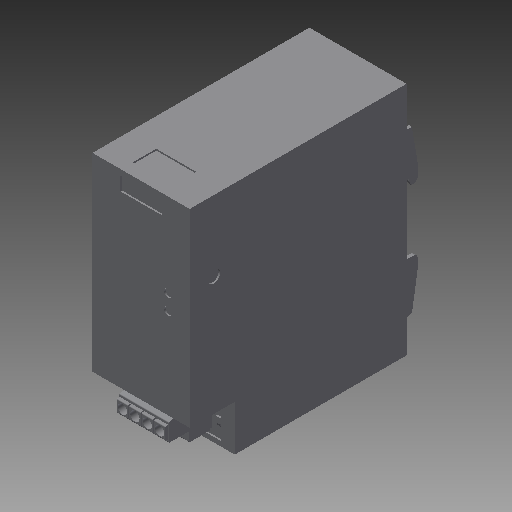
# Autodesk Inventor part: 172882
Saved by Autodesk Inventor 2019.3 (Build 233278000, 278)
## iProperties
Category: PARTsolutions
Company: MOELLER
Created: 2018-10-25
Part Number: 172882
Material: Generic
Catalog Web Link: www.cadenas.de
Description: PSG Power supply units-
Vendor: MOELLER
Document SubType Name: Modeling
Designer: psadmin
Manufacturer: MOELLER
Mass: 656.028 g
Surface Area: 554.305 cm^2
Volume: 656.028 cm^3
Density: 1 g/cm^3
Appearance: PSOLRGB-175-175-175
PSOL_IDENT_0: {$CADENAS_DATA\23d-libs\moeller\1589\1805\1806.prj},181 {VTYP=3D},{NB=172882},{LINA=172882},{NN=PSG
PSOL_IDENT_1: Power supply units},{DATE=04.10.2018 12:16:39},{GEOMDATE=04.10.2018 08:29:25},{VERSION=v181004082925
PSOL_IDENT_2: },{LINEID=10},{WBVAR=},{WBNUMERIC=}  {NB=172882},{LINA=172882},{KT=DUMMY},{PFOTO=2727pic-70.jpg},{PL
PSOL_IDENT_3: ID=172882},{DATA_SHEET=Data sheet},{MANUTYPEDESC=PSG60F24RM},{DESCSHORT=Power supply unit, 3-phase,
PSOL_IDENT_4: 100-240VAC/24VDC, 2.5A},{DESCLONG=Power supply unit, Product range: Power supplies PSG, Subrange: po
PSOL_IDENT_5: wer supply unit, Description: Power Boost via 1.5-fold rated operational current for 5 s, PELV (EN 6
PSOL_IDENT_6: 0204), SELV (EN 60950), Width: 50 mm, Height: 121 mm, Depth: 117.3 mm, Three-phase, Input voltage ra
PSOL_IDENT_7: nge: 320 - 600 V AC, (450 - 800 V DC), Nominal input voltage: 3 x 400 - 500 V AC, Rated output volta
PSOL_IDENT_8: ge: 24 V DC (± 2%), Rated output current: 2.5 A, Setting range for the output voltage: 24 - 28 V DC,
PSOL_IDENT_9: Rated output power: 60 W, Degree of Protection: IP20, Heat dissipation: 9.8 W},{EAN=4015081694709},
PSOL_IDENT_10: {ECLASS_8_1=27-04-90-02},{PACKAGED_WEIGHT=0.610},{DATA_SHEET_=http://datasheet.moeller.net/datasheet
PSOL_IDENT_11: .php?model=172882&locale=en_GB},{DATA_SHEET_ENG=http://datasheet.moeller.net/datasheet.php?model=172
PSOL_IDENT_12: 882&locale=en_GB},{DATA_SHEET_DEU=http://datasheet.moeller.net/datasheet.php?model=172882&locale=de_
PSOL_IDENT_13: DE}
NN: PSG Power supply units
NB: 172882
NBSYN: $PLID.
LINA: 172882
PFOTO: 2727pic-70.jpg
PLID: 172882
DATA_SHEET: Data sheet
MANUTYPEDESC: PSG60F24RM
DESCSHORT: Power supply unit, 3-phase, 100-240VAC/24VDC, 2.5A
DESCLONG: Power supply unit, Product range: Power supplies PSG, Subrange: power supply unit, Description: Power Boost via 1.5-fold rated operational current for 5 s, PELV (EN 60204), SELV (EN 60950), Width: 50 mm, Height: 121 mm, Depth: 117.3 mm, Three-phase, Input voltage range: 320 - 600 V AC, (450 - 800 V DC), Nominal input voltage: 3 x 400 - 500 V AC, Rated output voltage: 24 V DC (± 2%), Rated output current: 2.5 A, Setting range for the output voltage: 24 - 28 V DC, Rated output power: 60 W, Degree of Protection: IP20, Heat dissipation: 9.8 W
EAN: 4015081694709
ECLASS_8_1: 27-04-90-02
PACKAGED_WEIGHT: 0.61
SUPPLIER: MOELLER
ARTICLENO: 172882
BOMINFO: 172882
CREATOR: CADENAS GmbH
Title: 172882
Author: Cadenas PARTsolutions
Autodesk Inventor part; units mm, degrees
ref_plane "YZ Plane" through (0, 0, 0) normal (1, 0, 0) x (0, 1, 0)
ref_plane "XZ Plane" through (0, 0, 0) normal (0, 1, 0) x (-1, 0, 0)
ref_plane "XY Plane" through (0, 0, 0) normal (0, 0, 1) x (1, 0, 0)
sketch "Sketch_1" plane through (0, 0, 0) normal (1, 0, 0) x (0, 1, 0)
  line L0 (23.5, 23.2) -> (23.5, 0)
  line L1 (23.5, 0) -> (0, 0)
  line L2 (0, 0) -> (0, -88.4)
  line L3 (0, -88.4) -> (17, -88.4)
  line L4 (17, -88.4) -> (17, -89.3953)
  arc A0 (17, -89.3953) -> (18.6832, -91.37) centre (19, -89.3953) ccw
  line L5 (18.6832, -91.37) -> (35.7, -94.1)
  line L6 (35.7, -94.1) -> (40.7, -94.1)
  arc A1 (40.7, -94.1) -> (42.7, -92.1) centre (40.7, -92.1) ccw
  line L7 (42.7, -92.1) -> (42.7, -88.4)
  line L8 (42.7, -88.4) -> (78, -88.4)
  line L9 (78, -88.4) -> (78, -89.7)
  line L10 (78, -89.7) -> (77, -89.7)
  line L11 (77, -89.7) -> (74.7, -90.773)
  line L12 (74.7, -90.773) -> (74.7, -92.1)
  arc A2 (74.7, -92.1) -> (76.7, -94.1) centre (76.7, -92.1) ccw
  line L13 (76.7, -94.1) -> (83, -94.1)
  line L14 (83, -94.1) -> (100.5, -91.1)
  line L15 (100.5, -91.1) -> (100.5, -88.4)
  line L16 (100.5, -88.4) -> (121, -88.4)
  line L17 (121, -88.4) -> (121, 23.2)
  line L18 (121, 23.2) -> (23.5, 23.2)
  constraints: 38 end point, 6 point on circle, 3 centre point
extrude "Extrusion1" add sketch "Sketch_1" along normal blind 50
sketch "Sketch_2" plane through (0, 0, 0) normal (0, 1, 0) x (-1, 0, 0)
  line L0 (-1.6, -98.4) -> (-1.6, -88.4)
  line L1 (-1.6, -88.4) -> (-48.4, -88.4)
  line L2 (-48.4, -88.4) -> (-48.4, -98.4)
  line L3 (-48.4, -98.4) -> (-1.6, -98.4)
  constraints: 8 end point
extrude "Extrusion2" cut sketch "Sketch_2" along normal blind 120
sketch "Sketch_9" plane through (0, 0, 0) normal (0, 0, 1) x (1, 0, 0)
  line L0 (5.65, 22.3) -> (8.85, 22.3)
  line L1 (8.85, 22.3) -> (9.85, 21.3)
  line L2 (9.85, 21.3) -> (9.85, 18)
  line L3 (9.85, 18) -> (7.85, 18)
  line L4 (7.85, 18) -> (7.85, 19.5)
  arc A0 (7.85, 19.5) -> (6.85, 19.5) centre (7.35, 19.5) ccw
  line L5 (6.85, 19.5) -> (6.85, 12.5)
  line L6 (6.85, 12.5) -> (9.85, 12.5)
  line L7 (9.85, 12.5) -> (9.85, 8)
  line L8 (9.85, 8) -> (7.85, 8)
  line L9 (7.85, 8) -> (7.85, 9.5)
  arc A1 (7.85, 9.5) -> (6.85, 9.5) centre (7.35, 9.5) ccw
  line L10 (6.85, 9.5) -> (6.85, 2.5)
  line L11 (6.85, 2.5) -> (43.15, 2.5)
  line L12 (43.15, 2.5) -> (43.15, 9.5)
  arc A2 (43.15, 9.5) -> (42.15, 9.5) centre (42.65, 9.5) ccw
  line L13 (42.15, 9.5) -> (42.15, 8)
  line L14 (42.15, 8) -> (40.15, 8)
  line L15 (40.15, 8) -> (40.15, 12.5)
  line L16 (40.15, 12.5) -> (43.15, 12.5)
  line L17 (43.15, 12.5) -> (43.15, 19.5)
  arc A3 (43.15, 19.5) -> (42.15, 19.5) centre (42.65, 19.5) ccw
  line L18 (42.15, 19.5) -> (42.15, 18)
  line L19 (42.15, 18) -> (40.15, 18)
  line L20 (40.15, 18) -> (40.15, 21.3)
  line L21 (40.15, 21.3) -> (41.15, 22.3)
  line L22 (41.15, 22.3) -> (44.35, 22.3)
  line L23 (44.35, 22.3) -> (44.35, 23.484)
  line L24 (44.35, 23.484) -> (5.65, 23.484)
  line L25 (5.65, 23.484) -> (5.65, 22.3)
  line L26 (12.3, 20.65) -> (12.3, 5.6)
  line L27 (12.3, 5.6) -> (37.7, 5.6)
  line L28 (37.7, 5.6) -> (37.7, 20.65)
  line L29 (37.7, 20.65) -> (12.3, 20.65)
  constraints: 60 end point, 8 point on circle, 4 centre point
extrude "Extrusion3" cut sketch "Sketch_9" against normal blind 0.8
sketch "Sketch_10" plane through (25, 0, 0) normal (1, 0, 0) x (0, 0, -1)
  line L0 (0, 19.5) -> (0, 18)
  line L1 (0, 18) -> (0.8, 18)
  line L2 (0.8, 18) -> (0, 19.5)
  constraints: 6 end point
extrude "Extrusion4" cut sketch "Sketch_10" along normal mid plane 36
sketch "Sketch_11" plane through (25, 0, 0) normal (1, 0, 0) x (0, 0, -1)
  line L0 (0, 9.5) -> (0, 8)
  line L1 (0, 8) -> (0.8, 8)
  line L2 (0.8, 8) -> (0, 9.5)
  constraints: 6 end point
extrude "Extrusion5" cut sketch "Sketch_11" along normal mid plane 36
sketch "Sketch_12" plane through (25, 0, 0) normal (1, 0, 0) x (0, 0, -1)
  line L0 (0, 9.5) -> (0, 8)
  line L1 (0, 8) -> (0.8, 8)
  line L2 (0.8, 8) -> (0, 9.5)
  constraints: 6 end point
extrude "Extrusion6" add sketch "Sketch_12" along normal mid plane 25.4
sketch "Sketch_13" plane through (25, 0, 0) normal (1, 0, 0) x (0, 0, -1)
  line L0 (0, 19.5) -> (0, 18)
  line L1 (0, 18) -> (0.8, 18)
  line L2 (0.8, 18) -> (0, 19.5)
  constraints: 6 end point
extrude "Extrusion7" add sketch "Sketch_13" along normal mid plane 25.4
sketch "Sketch_3" plane through (25, 0, 0) normal (1, 0, 0) x (0, 0, -1)
  line L0 (-23.2, 17.3) -> (-23.2, 11.8)
  arc A0 (-23.2, 11.8) -> (-22.7, 11.3) centre (-22.7, 11.8) ccw
  line L1 (-22.7, 11.3) -> (-21.7, 11.3)
  line L2 (-21.7, 11.3) -> (-21.7, 10.3)
  arc A1 (-21.7, 10.3) -> (-21.2, 9.8) centre (-21.2, 10.3) ccw
  line L3 (-21.2, 9.8) -> (-11.25, 9.8)
  line L4 (-11.25, 9.8) -> (-11.25, 5.3)
  arc A2 (-11.25, 5.3) -> (-10.75, 4.8) centre (-10.75, 5.3) ccw
  line L5 (-10.75, 4.8) -> (-0.25, 4.8)
  line L6 (-0.25, 4.8) -> (-0.25, 5.6)
  line L7 (-0.25, 5.6) -> (0, 5.6)
  line L8 (0, 5.6) -> (0, 20.65)
  line L9 (0, 20.65) -> (-11.25, 20.65)
  line L10 (-11.25, 20.65) -> (-21.272, 19.1912)
  arc A3 (-21.272, 19.1912) -> (-21.7, 18.6964) centre (-21.2, 18.6964) ccw
  line L11 (-21.7, 18.6964) -> (-21.7, 17.8)
  line L12 (-21.7, 17.8) -> (-22.7, 17.8)
  arc A4 (-22.7, 17.8) -> (-23.2, 17.3) centre (-22.7, 17.3) ccw
  constraints: 26 end point, 10 point on circle, 5 centre point
extrude "Extrusion8" add sketch "Sketch_3" along normal mid plane 25.4
sketch "Sketch_4" plane through (0, 0, 0) normal (0, 1, 0) x (-1, 0, 0)
  line L0 (-11.3, 31.7) -> (-38.7, 31.7)
  line L1 (-38.7, 31.7) -> (-38.7, 21.7)
  line L2 (-38.7, 21.7) -> (-37.425, 21.7)
  line L3 (-37.425, 21.7) -> (-37.425, 23.2)
  line L4 (-37.425, 23.2) -> (-31.625, 23.2)
  line L5 (-31.625, 23.2) -> (-31.625, 21.7)
  line L6 (-31.625, 21.7) -> (-31.075, 21.7)
  line L7 (-31.075, 21.7) -> (-31.075, 23.2)
  line L8 (-31.075, 23.2) -> (-25.275, 23.2)
  line L9 (-25.275, 23.2) -> (-25.275, 21.7)
  line L10 (-25.275, 21.7) -> (-24.725, 21.7)
  line L11 (-24.725, 21.7) -> (-24.725, 23.2)
  line L12 (-24.725, 23.2) -> (-18.925, 23.2)
  line L13 (-18.925, 23.2) -> (-18.925, 21.7)
  line L14 (-18.925, 21.7) -> (-18.375, 21.7)
  line L15 (-18.375, 21.7) -> (-18.375, 23.2)
  line L16 (-18.375, 23.2) -> (-12.575, 23.2)
  line L17 (-12.575, 23.2) -> (-12.575, 21.7)
  line L18 (-12.575, 21.7) -> (-11.3, 21.7)
  line L19 (-11.3, 21.7) -> (-11.3, 31.7)
  constraints: 40 end point
extrude "Extrusion9" cut sketch "Sketch_4" along normal blind 20
sketch "Sketch10" plane through (12.575, 11.8, 23.2) normal (0, 0, 1) x (1, 0, 0)
  point P0 (2.9, 2.75)
hole "Hole1" at (15.475, 14.55, 23.2) direction (0, 0, -1) diameter 4.85 depth 4.91
sketch "Sketch11" plane through (18.925, 11.8, 23.2) normal (0, 0, 1) x (1, 0, 0)
  point P0 (2.9, 2.75)
hole "Hole2" at (21.825, 14.55, 23.2) direction (0, 0, -1) diameter 4.85 depth 4.91
sketch "Sketch12" plane through (25.275, 11.8, 23.2) normal (0, 0, 1) x (1, 0, 0)
  point P0 (2.9, 2.75)
hole "Hole3" at (28.175, 14.55, 23.2) direction (0, 0, -1) diameter 4.85 depth 4.91
sketch "Sketch13" plane through (31.625, 11.8, 23.2) normal (0, 0, 1) x (1, 0, 0)
  point P0 (2.9, 2.75)
hole "Hole4" at (34.525, 14.55, 23.2) direction (0, 0, -1) diameter 4.85 depth 4.91
sketch "Sketch14" plane through (0, 23.5, 23.2) normal (0, 0, 1) x (1, 0, 0)
  point P0 (38.9, 54.4)
hole "Hole5" at (38.9, 77.9, 23.2) direction (0, 0, -1) diameter 4 depth 0.8
sketch "Sketch15" plane through (0, 23.5, 23.2) normal (0, 0, 1) x (1, 0, 0)
  point P0 (38.9, 46.4)
hole "Hole6" at (38.9, 69.9, 23.2) direction (0, 0, -1) diameter 4 depth 0.8
sketch "Sketch_18" plane through (0, 0, 23.2) normal (0, 0, 1) x (1, 0, 0)
  line L0 (14.33, 118.05) -> (14.33, 111.05)
  line L1 (14.33, 111.05) -> (35.67, 111.05)
  line L2 (35.67, 111.05) -> (35.67, 118.05)
  line L3 (35.67, 118.05) -> (14.33, 118.05)
  constraints: 8 end point
extrude "Extrusion10" cut sketch "Sketch_18" against normal blind 0.8
sketch "Sketch_19" plane through (0, 121, 0) normal (0, 1, 0) x (1, 0, 0)
  line L0 (14.58, -17.2) -> (35.06, -17.2)
  line L1 (35.06, -17.2) -> (35.06, -4.95)
  line L2 (35.06, -4.95) -> (14.58, -4.95)
  line L3 (14.58, -4.95) -> (14.58, -17.2)
  constraints: 8 end point
extrude "Extrusion11" cut sketch "Sketch_19" against normal blind 0.8
sketch "Sketch_20" plane through (0, 17, 0) normal (0, 1, 0) x (1, 0, 0)
  line L0 (13.557, 88.4) -> (15.182, 88.4)
  line L1 (15.182, 88.4) -> (15.3929, 89.6)
  line L2 (15.3929, 89.6) -> (34.6071, 89.6)
  line L3 (34.6071, 89.6) -> (34.818, 88.4)
  line L4 (34.818, 88.4) -> (36.443, 88.4)
  line L5 (36.443, 88.4) -> (36.1835, 89.8769)
  arc A0 (36.1835, 89.8769) -> (34.6076, 91.2) centre (34.6076, 89.6) ccw
  line L6 (34.6076, 91.2) -> (15.3924, 91.2)
  arc A1 (15.3924, 91.2) -> (13.8165, 89.8769) centre (15.3924, 89.6) ccw
  line L7 (13.8165, 89.8769) -> (13.557, 88.4)
  constraints: 16 end point, 4 point on circle, 2 centre point
extrude "Extrusion12" add sketch "Sketch_20" along normal blind 25.7
sketch "Sketch_21" plane through (0, 17, 0) normal (0, 1, 0) x (1, 0, 0)
  line L0 (18.249, 93.5) -> (18.249, 88.5)
  line L1 (18.249, 88.5) -> (31.751, 88.5)
  line L2 (31.751, 88.5) -> (31.751, 93.5)
  line L3 (31.751, 93.5) -> (18.249, 93.5)
  constraints: 8 end point
extrude "Extrusion13" cut sketch "Sketch_21" along normal blind 25.7
sketch "Sketch_22" plane through (25, 0, 0) normal (1, 0, 0) x (0, 0, -1)
  line L0 (88.4, 33.7) -> (88.4, 23)
  line L1 (88.4, 23) -> (93.4, 23)
  line L2 (93.4, 23) -> (93.4, 33.7)
  line L3 (93.4, 33.7) -> (88.4, 33.7)
  constraints: 8 end point
extrude "Extrusion14" cut sketch "Sketch_22" along normal mid plane 25.7
sketch "Sketch_24" plane through (0, 0.5, 0) normal (0, 1, 0) x (1, 0, 0)
  line L0 (7.5, 90.1) -> (7.5, 88.4)
  line L1 (7.5, 88.4) -> (42.5, 88.4)
  line L2 (42.5, 88.4) -> (42.5, 90.1)
  arc A0 (42.5, 90.1) -> (40.5, 92.1) centre (40.5, 90.1) ccw
  line L3 (40.5, 92.1) -> (9.5, 92.1)
  arc A1 (9.5, 92.1) -> (7.5, 90.1) centre (9.5, 90.1) ccw
  constraints: 8 end point, 4 point on circle, 2 centre point
extrude "Extrusion15" add sketch "Sketch_24" along normal blind 1.6
sketch "Sketch_23" plane through (0, 0.5, 0) normal (0, 1, 0) x (1, 0, 0)
  line L0 (15.2, 93.6) -> (15.2, 92.1)
  line L1 (15.2, 92.1) -> (20.9, 92.1)
  arc A0 (22.9, 90.1) -> (20.9, 92.1) centre (20.9, 90.1) ccw
  arc A1 (22.4, 89.6) -> (22.9, 90.1) centre (22.4, 90.1) ccw
  line L2 (22.4, 89.6) -> (15.2, 89.6)
  line L3 (15.2, 89.6) -> (15.2, 88.4)
  line L4 (15.2, 88.4) -> (34.8, 88.4)
  line L5 (34.8, 88.4) -> (34.8, 89.6)
  line L6 (34.8, 89.6) -> (27.6, 89.6)
  arc A2 (27.1, 90.1) -> (27.6, 89.6) centre (27.6, 90.1) ccw
  arc A3 (29.1, 92.1) -> (27.1, 90.1) centre (29.1, 90.1) ccw
  line L7 (29.1, 92.1) -> (34.8, 92.1)
  line L8 (34.8, 92.1) -> (34.8, 93.6)
  line L9 (34.8, 93.6) -> (15.2, 93.6)
  constraints: 20 end point, 8 point on circle, 4 centre point
extrude "Extrusion16" cut sketch "Sketch_23" along normal blind 1.6
sketch "Sketch_25" plane through (0, 0, -88.4) normal (0, 0, 1) x (1, 0, 0)
  line L0 (15.6, 25.5) -> (15.6, 12.5)
  arc A0 (15.6, 12.5) -> (16.1, 12) centre (16.1, 12.5) ccw
  line L1 (16.1, 12) -> (17.9, 12)
  arc A1 (18.4, 11.5) -> (17.9, 12) centre (17.9, 11.5) ccw
  line L2 (18.4, 11.5) -> (18.4, 10)
  arc A2 (17.9, 9.5) -> (18.4, 10) centre (17.9, 10) ccw
  line L3 (17.9, 9.5) -> (16.1, 9.5)
  arc A3 (16.1, 9.5) -> (15.6, 9) centre (16.1, 9) ccw
  line L4 (15.6, 9) -> (15.6, -2.5)
  arc A4 (15.6, -2.5) -> (18.1, -5) centre (18.1, -2.5) ccw
  line L5 (18.1, -5) -> (32.1, -5)
  arc A5 (32.1, -5) -> (34.6, -2.5) centre (32.1, -2.5) ccw
  line L6 (34.6, -2.5) -> (34.6, 9)
  arc A6 (34.6, 9) -> (34.1, 9.5) centre (34.1, 9) ccw
  line L7 (34.1, 9.5) -> (32.3, 9.5)
  arc A7 (31.8, 10) -> (32.3, 9.5) centre (32.3, 10) ccw
  line L8 (31.8, 10) -> (31.8, 11.5)
  arc A8 (32.3, 12) -> (31.8, 11.5) centre (32.3, 11.5) ccw
  line L9 (32.3, 12) -> (34.1, 12)
  arc A9 (34.1, 12) -> (34.6, 12.5) centre (34.1, 12.5) ccw
  line L10 (34.6, 12.5) -> (34.6, 25.5)
  arc A10 (34.6, 25.5) -> (34.1, 26) centre (34.1, 25.5) ccw
  line L11 (34.1, 26) -> (32.3, 26)
  arc A11 (31.8, 26.5) -> (32.3, 26) centre (32.3, 26.5) ccw
  line L12 (31.8, 26.5) -> (31.8, 32.5)
  arc A12 (32.3, 33) -> (31.8, 32.5) centre (32.3, 32.5) ccw
  line L13 (32.3, 33) -> (34.1, 33)
  arc A13 (34.1, 33) -> (34.6, 33.5) centre (34.1, 33.5) ccw
  line L14 (34.6, 33.5) -> (34.6, 42)
  line L15 (34.6, 42) -> (15.6, 42)
  line L16 (15.6, 42) -> (15.6, 33.5)
  arc A14 (15.6, 33.5) -> (16.1, 33) centre (16.1, 33.5) ccw
  line L17 (16.1, 33) -> (17.9, 33)
  arc A15 (18.4, 32.5) -> (17.9, 33) centre (17.9, 32.5) ccw
  line L18 (18.4, 32.5) -> (18.4, 26.5)
  arc A16 (17.9, 26) -> (18.4, 26.5) centre (17.9, 26.5) ccw
  line L19 (17.9, 26) -> (16.1, 26)
  arc A17 (16.1, 26) -> (15.6, 25.5) centre (16.1, 25.5) ccw
  arc A18 (21.9, 1.5) -> (21.9, -1.5) centre (21.9, 0) ccw
  line L20 (21.9, -1.5) -> (27.9, -1.5)
  arc A19 (27.9, -1.5) -> (27.9, 1.5) centre (27.9, 0) ccw
  line L21 (27.9, 1.5) -> (21.9, 1.5)
  arc A20 (20.35, 21.5) -> (20.85, 21) centre (20.85, 21.5) ccw
  line L22 (20.85, 21) -> (20.85, 6.5)
  line L23 (20.85, 6.5) -> (29.35, 6.5)
  line L24 (29.35, 6.5) -> (29.35, 21)
  arc A21 (29.35, 21) -> (29.85, 21.5) centre (29.35, 21.5) ccw
  line L25 (29.85, 21.5) -> (29.85, 22)
  arc A22 (29.85, 22) -> (29.35, 22.5) centre (29.35, 22) ccw
  line L26 (29.35, 22.5) -> (28.85, 22.5)
  arc A23 (28.35, 23) -> (28.85, 22.5) centre (28.85, 23) ccw
  line L27 (28.35, 23) -> (28.35, 29.767)
  line L28 (28.35, 29.767) -> (21.85, 29.767)
  line L29 (21.85, 29.767) -> (21.85, 23)
  arc A24 (21.35, 22.5) -> (21.85, 23) centre (21.35, 23) ccw
  line L30 (21.35, 22.5) -> (20.85, 22.5)
  arc A25 (20.85, 22.5) -> (20.35, 22) centre (20.85, 22) ccw
  line L31 (20.35, 22) -> (20.35, 21.5)
  constraints: 64 end point, 52 point on circle, 26 centre point
extrude "Extrusion17" add sketch "Sketch_25" against normal blind 1
sketch "Sketch_26" plane through (0, 6.5, 0) normal (0, 1, 0) x (1, 0, 0)
  arc A0 (20.85, 88.4) -> (21.85, 89.4) centre (20.85, 89.4) ccw
  line L0 (21.85, 89.4) -> (21.85, 91.4)
  line L1 (21.85, 91.4) -> (20.85, 91.4)
  line L2 (20.85, 91.4) -> (20.85, 88.4)
  constraints: 6 end point, 2 point on circle, 1 centre point
sketch "Sketch_27" plane through (0, 6.5, 0) normal (0, 1, 0) x (1, 0, 0)
  arc A0 (28.35, 89.4) -> (29.35, 88.4) centre (29.35, 89.4) ccw
  line L0 (29.35, 88.4) -> (29.35, 91.4)
  line L1 (29.35, 91.4) -> (28.35, 91.4)
  line L2 (28.35, 91.4) -> (28.35, 89.4)
  constraints: 6 end point, 2 point on circle, 1 centre point
extrude "Extrusion18" add sketch "Sketch_27" along normal blind 14.5
extrude "Extrusion19" add sketch "Sketch_26" along normal blind 14.5
sketch "Sketch_30" plane through (25, 0, 0) normal (1, 0, 0) x (0, 0, -1)
  line L0 (90.4, 5.5) -> (95.4, 5.5)
  line L1 (95.4, 5.5) -> (95.4, 22)
  line L2 (95.4, 22) -> (90.4, 22)
  line L3 (90.4, 22) -> (90.4, 21)
  line L4 (90.4, 21) -> (90.9, 21)
  arc A0 (91.4, 20.5) -> (90.9, 21) centre (90.9, 20.5) ccw
  line L5 (91.4, 20.5) -> (91.4, 7)
  arc A1 (90.9, 6.5) -> (91.4, 7) centre (90.9, 7) ccw
  line L6 (90.9, 6.5) -> (90.4, 6.5)
  line L7 (90.4, 6.5) -> (90.4, 5.5)
  constraints: 16 end point, 4 point on circle, 2 centre point
extrude "Extrusion20" cut sketch "Sketch_30" along normal mid plane 10
sketch "Sketch_31" plane through (0, 0, -89.4) normal (0, 0, 1) x (1, 0, 0)
  arc A0 (21.15, 37) -> (21.9, 36.25) centre (21.9, 37) ccw
  line L0 (21.9, 36.25) -> (27.9, 36.25)
  arc A1 (27.9, 36.25) -> (28.65, 37) centre (27.9, 37) ccw
  arc A2 (28.65, 37) -> (27.9, 37.75) centre (27.9, 37) ccw
  line L1 (27.9, 37.75) -> (21.9, 37.75)
  arc A3 (21.9, 37.75) -> (21.15, 37) centre (21.9, 37) ccw
  constraints: 8 point on circle, 4 centre point, 4 end point
extrude "Extrusion21" add sketch "Sketch_31" against normal blind 0.5
sketch "Sketch_32" plane through (25, 0, 0) normal (1, 0, 0) x (0, 0, -1)
  line L0 (82.9551, 62.6899) -> (83.2925, 61.2284)
  line L1 (83.2925, 61.2284) -> (88.9212, 62.5278)
  arc A0 (88.9212, 62.5278) -> (90.1, 64.0099) centre (88.579, 64.0099) ccw
  line L2 (90.1, 64.0099) -> (90.1, 69.8)
  line L3 (90.1, 69.8) -> (88.6, 69.8)
  line L4 (88.6, 69.8) -> (88.6, 63.9932)
  line L5 (88.6, 63.9932) -> (82.9551, 62.6899)
  constraints: 12 end point, 2 point on circle, 1 centre point
extrude "Extrusion22" add sketch "Sketch_32" along normal mid plane 35.4
sketch "Sketch_33" plane through (25, 0, 0) normal (1, 0, 0) x (0, 0, -1)
  line L0 (88.4, 61.3) -> (98.4, 61.3)
  line L1 (98.4, 61.3) -> (98.4, 71.3)
  line L2 (98.4, 71.3) -> (88.4, 71.3)
  line L3 (88.4, 71.3) -> (88.4, 61.3)
  constraints: 8 end point
extrude "Extrusion23" cut sketch "Sketch_33" along normal mid plane 25.4
sketch "Sketch_34" plane through (0, 0, -88.4) normal (0, 0, 1) x (1, 0, 0)
  circle A0 centre (7, 84.5) radius 2.6
  circle A1 centre (7, 84.5) radius 1.25
  constraints: 2 centre point
extrude "Extrusion24" add sketch "Sketch_34" against normal blind 1.4
sketch "Sketch_35" plane through (0, 0, -88.4) normal (0, 0, 1) x (1, 0, 0)
  circle A0 centre (43, 84.5) radius 2.6
  circle A1 centre (43, 84.5) radius 1.25
  constraints: 2 centre point
extrude "Extrusion25" add sketch "Sketch_35" against normal blind 1.4
sketch "Sketch_36" plane through (0, 0, -88.4) normal (0, 0, 1) x (1, 0, 0)
  circle A0 centre (14, 74.5) radius 1
  constraints: 1 centre point
extrude "Extrusion26" add sketch "Sketch_36" against normal blind 0.8
sketch "Sketch_37" plane through (0, 0, -88.4) normal (0, 0, 1) x (1, 0, 0)
  circle A0 centre (36, 74.5) radius 1
  constraints: 1 centre point
extrude "Extrusion27" add sketch "Sketch_37" against normal blind 0.8
sketch "Sketch_38" plane through (0, 0, -88.4) normal (0, 0, 1) x (1, 0, 0)
  circle A0 centre (7, 14.5) radius 2.6
  circle A1 centre (7, 14.5) radius 1.25
  constraints: 2 centre point
sketch "Sketch_39" plane through (0, 0, -88.4) normal (0, 0, 1) x (1, 0, 0)
  circle A0 centre (43, 14.5) radius 2.6
  circle A1 centre (43, 14.5) radius 1.25
  constraints: 2 centre point
extrude "Extrusion28" add sketch "Sketch_38" against normal blind 1.4
extrude "Extrusion29" add sketch "Sketch_39" against normal blind 1.4
sketch "Sketch_40" plane through (25, 0, 0) normal (1, 0, 0) x (0, 0, -1)
  line L0 (-10.25, 8.5406) -> (-10.25, 0)
  line L1 (-10.25, 0) -> (-1.25, 0)
  line L2 (-1.25, 0) -> (-1.25, 6.757)
  line L3 (-1.25, 6.757) -> (-4.15, 9.7995)
  line L4 (-4.15, 9.7995) -> (-4.15, 10.8)
  line L5 (-4.15, 10.8) -> (-9.05, 10.8)
  line L6 (-9.05, 10.8) -> (-9.05, 9.7995)
  line L7 (-9.05, 9.7995) -> (-10.25, 8.5406)
  constraints: 16 end point
extrude "Extrusion30" cut sketch "Sketch_40" along normal mid plane 23
sketch "Sketch_41" plane through (0, 0, 0.8) normal (0, 0, 1) x (1, 0, 0)
  line L0 (12.875, 10.8) -> (18.025, 10.8)
  line L1 (18.025, 10.8) -> (18.025, 7.21)
  line L2 (18.025, 7.21) -> (17.153, 5.6239)
  line L3 (17.153, 5.6239) -> (17.153, 4.8)
  line L4 (17.153, 4.8) -> (20.097, 4.8)
  line L5 (20.097, 4.8) -> (20.097, 5.6239)
  line L6 (20.097, 5.6239) -> (19.225, 7.21)
  line L7 (19.225, 7.21) -> (19.225, 10.8)
  line L8 (19.225, 10.8) -> (24.375, 10.8)
  line L9 (24.375, 10.8) -> (24.375, 7.21)
  line L10 (24.375, 7.21) -> (23.503, 5.6239)
  line L11 (23.503, 5.6239) -> (23.503, 4.8)
  line L12 (23.503, 4.8) -> (26.447, 4.8)
  line L13 (26.447, 4.8) -> (26.447, 5.6239)
  line L14 (26.447, 5.6239) -> (25.575, 7.21)
  line L15 (25.575, 7.21) -> (25.575, 10.8)
  line L16 (25.575, 10.8) -> (30.725, 10.8)
  line L17 (30.725, 10.8) -> (30.725, 7.21)
  line L18 (30.725, 7.21) -> (29.853, 5.6239)
  line L19 (29.853, 5.6239) -> (29.853, 4.8)
  line L20 (29.853, 4.8) -> (32.797, 4.8)
  line L21 (32.797, 4.8) -> (32.797, 5.6239)
  line L22 (32.797, 5.6239) -> (31.925, 7.21)
  line L23 (31.925, 7.21) -> (31.925, 10.8)
  line L24 (31.925, 10.8) -> (37.075, 10.8)
  line L25 (37.075, 10.8) -> (37.075, 11.5)
  line L26 (37.075, 11.5) -> (12.875, 11.5)
  line L27 (12.875, 11.5) -> (12.875, 10.8)
  constraints: 56 end point
extrude "Extrusion31" add sketch "Sketch_41" along normal blind 9.7
sketch "Sketch38" plane through (50, 0, 0) normal (1, 0, 0) x (0, 0, -1)
  point P0 (-10.7, 84.8)
hole "Hole7" at (50, 84.8, 10.7) direction (-1, 0, 0) diameter 6.5 depth 0.8
sketch "Sketch39" plane through (0, 0, 0) normal (-1, 0, 0) x (0, 0, 1)
  point P0 (9.5, 67.7)
hole "Hole8" at (0, 67.7, 9.5) direction (1, 0, 0) diameter 6.5 depth 0.8
sketch "Sketch_46" plane through (0, 0, 0) normal (1, 0, 0) x (0, 1, 0)
  line L0 (43.9, -1.6) -> (32.9, -1.6)
  line L1 (32.9, -1.6) -> (32.9, -3.6)
  line L2 (32.9, -3.6) -> (43.9, -3.6)
  line L3 (43.9, -3.6) -> (43.9, -1.6)
  constraints: 8 end point
extrude "Extrusion32" cut sketch "Sketch_46" along normal blind 0.8
sketch "Sketch_47" plane through (0, 0, 0) normal (1, 0, 0) x (0, 1, 0)
  line L0 (104.2, 7.4) -> (93.2, 7.4)
  line L1 (93.2, 7.4) -> (93.2, 5.4)
  line L2 (93.2, 5.4) -> (104.2, 5.4)
  line L3 (104.2, 5.4) -> (104.2, 7.4)
  constraints: 8 end point
extrude "Extrusion33" cut sketch "Sketch_47" along normal blind 0.8
sketch "Sketch_42" plane through (25, 0, 0) normal (1, 0, 0) x (0, 0, -1)
  line L0 (88.4, 42) -> (89.601, 42)
  arc A0 (89.601, 42) -> (90.5858, 42.8264) centre (89.601, 43) ccw
  line L1 (90.5858, 42.8264) -> (91.0037, 45.1963)
  line L2 (91.0037, 45.1963) -> (94.278, 41.2942)
  line L3 (94.278, 41.2942) -> (95.044, 41.937)
  line L4 (95.044, 41.937) -> (91.7697, 45.8391)
  arc A1 (91.7697, 45.8391) -> (90.0189, 45.37) centre (91.0037, 45.1963) ccw
  line L5 (90.0189, 45.37) -> (89.601, 43)
  line L6 (89.601, 43) -> (89.4, 43)
  arc A2 (89.4, 43) -> (88.4, 42) centre (89.4, 42) ccw
  constraints: 14 end point, 6 point on circle, 3 centre point
extrude "Extrusion34" add sketch "Sketch_42" along normal mid plane 13
sketch "Sketch_44" plane through (18.5, 45.8391, -91.7697) normal (0, 0.6428, -0.766) x (0, -0.766, -0.6428)
  line L0 (4.095, -13) -> (7.095, -13)
  line L1 (7.095, -13) -> (7.095, 0)
  line L2 (7.095, 0) -> (4.095, 0)
  arc A0 (5.095, -1) -> (4.095, 0) centre (4.095, -1) ccw
  line L3 (5.095, -1) -> (5.095, -12)
  arc A1 (4.095, -13) -> (5.095, -12) centre (4.095, -12) ccw
  constraints: 8 end point, 4 point on circle, 2 centre point
extrude "Extrusion35" cut sketch "Sketch_44" along normal mid plane 2
sketch "Sketch_48" plane through (25, 0, 0) normal (1, 0, 0) x (0, 0, -1)
  line L0 (88.4, 8.1) -> (88.4, 6.5)
  line L1 (88.4, 6.5) -> (90.1, 6.5)
  arc A0 (90.1, 6.5) -> (91.7, 8.1) centre (90.1, 8.1) ccw
  line L2 (91.7, 8.1) -> (88.4, 8.1)
  constraints: 6 end point, 2 point on circle, 1 centre point
extrude "Extrusion36" add sketch "Sketch_48" along normal mid plane 6
sketch "Sketch_49" plane through (0, 0, -91.7) normal (0, 0, 1) x (1, 0, 0)
  line L0 (22, 10.5) -> (22, 8.1)
  line L1 (22, 8.1) -> (28, 8.1)
  line L2 (28, 8.1) -> (28, 10.5)
  line L3 (28, 10.5) -> (26.5, 10.5)
  line L4 (26.5, 10.5) -> (26.5, 12.8)
  arc A0 (26.5, 12.8) -> (26, 13.3) centre (26, 12.8) ccw
  line L5 (26, 13.3) -> (24, 13.3)
  arc A1 (24, 13.3) -> (23.5, 12.8) centre (24, 12.8) ccw
  line L6 (23.5, 12.8) -> (23.5, 10.5)
  line L7 (23.5, 10.5) -> (22, 10.5)
  constraints: 16 end point, 4 point on circle, 2 centre point
extrude "Extrusion37" add sketch "Sketch_49" along normal blind 1
sketch "Sketch_51" plane through (21.85, 0, 0) normal (1, 0, 0) x (0, 0, -1)
  line L0 (88.4, 28.7347) -> (89.4, 28.7347)
  line L1 (89.4, 28.7347) -> (90.4, 28.4668)
  line L2 (90.4, 28.4668) -> (90.4, 22.46)
  line L3 (90.4, 22.46) -> (91.4, 22.46)
  line L4 (91.4, 22.46) -> (91.4, 28.46)
  arc A0 (91.4, 28.46) -> (90.6588, 29.4327) centre (90.4, 28.4668) ccw
  line L5 (90.6588, 29.4327) -> (89.4, 29.77)
  line L6 (89.4, 29.77) -> (88.4, 29.77)
  line L7 (88.4, 29.77) -> (88.4, 28.7347)
  constraints: 16 end point, 2 point on circle, 1 centre point
extrude "Extrusion38" add sketch "Sketch_51" along normal blind 6.5
sketch "Sketch_52" plane through (0, 0, -91.4) normal (0, 0, 1) x (1, 0, 0)
  line L0 (21.35, 21.464) -> (28.85, 21.464)
  line L1 (28.85, 21.464) -> (28.85, 25.664)
  line L2 (28.85, 25.664) -> (26.6, 25.664)
  line L3 (26.6, 25.664) -> (26.6, 23.701)
  arc A0 (26.1, 23.201) -> (26.6, 23.701) centre (26.1, 23.701) ccw
  line L4 (26.1, 23.201) -> (24.1, 23.201)
  arc A1 (23.6, 23.701) -> (24.1, 23.201) centre (24.1, 23.701) ccw
  line L5 (23.6, 23.701) -> (23.6, 25.664)
  line L6 (23.6, 25.664) -> (21.35, 25.664)
  line L7 (21.35, 25.664) -> (21.35, 21.464)
  constraints: 16 end point, 4 point on circle, 2 centre point
extrude "Extrusion39" cut sketch "Sketch_52" along normal mid plane 3
sketch "Sketch_50" plane through (25, 0, 0) normal (1, 0, 0) x (0, 0, -1)
  line L0 (90.9, 25.35) -> (90.9, 10.5)
  line L1 (90.9, 10.5) -> (88.5, 10.5)
  line L2 (88.5, 10.5) -> (88.5, 25.35)
  line L3 (88.5, 25.35) -> (90.9, 25.35)
  line L4 (90.9, 25.35) -> (90.9, 10.5)
  constraints: 10 end point
revolve "Revolution1" add sketch "Sketch_50" angle 360 about axis through (25, 25.35, -90.9) along (0, 1, 0)
body "Solid1"
